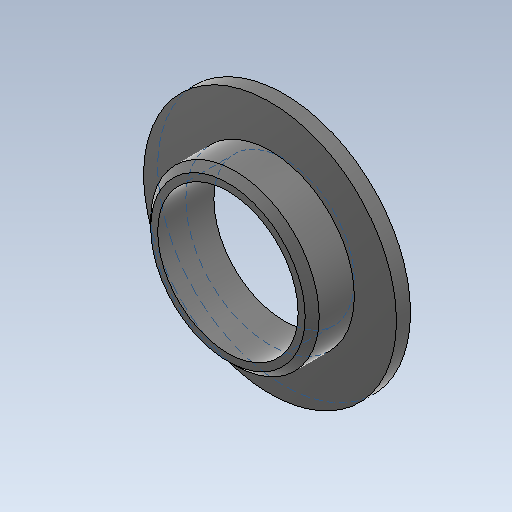
# Autodesk Inventor part: オイレスw5f10-12a
Saved by Autodesk Inventor 2020 (Build 240168000, 168)
## iProperties
Created: 2020-02-11
Part Number: オイレスw5f10-12a
Material: アセタール樹脂、黒
Document SubType Name: Modeling
Designer: happy
Density: 1.425 g/cm^3
Appearance: 滑らか - 黒
Mass: 0.391904 g
Surface Area: 6.35801 cm^2
Volume: 0.27502 cm^3
Author: happy
Autodesk Inventor part; units mm, degrees
ref_plane "YZ Plane" through (0, 0, 0) normal (1, 0, 0) x (0, 1, 0)
ref_plane "XZ Plane" through (0, 0, 0) normal (0, 1, 0) x (-1, 0, 0)
ref_plane "XY Plane" through (0, 0, 0) normal (0, 0, 1) x (1, 0, 0)
sketch "スケッチ1" plane through (0, 0, 0) normal (0, 0, 1) x (1, 0, 0)
  circle A0 centre (0, 0) radius 5
  circle A1 centre (0, 0) radius 9
  dimension "d0" = 10
  dimension "d1" = 18
  constraints: 2 centre point, 2 coincident
  measures "d0" diameter of A0
  measures "d1" diameter of A1
extrude "押し出し1" add sketch "スケッチ1" along normal blind 1
sketch "スケッチ2" plane through (0, 0, 1) normal (0, 0, 1) x (1, 0, 0)
  circle A0 centre (0, 0) radius 6
  circle A1 centre (0, 0) radius 9 projected
  circle A2 centre (0, 0) radius 5 projected
  dimension "d4" = 12
  constraints: 1 centre point, 1 coincident
  measures "d4" diameter of A0
extrude "押し出し2" add sketch "スケッチ2" along normal blind 3 contours A0
chamfer "面取り1" distance 0.5 angle 45 1 edges at (-6, 0, 4)
